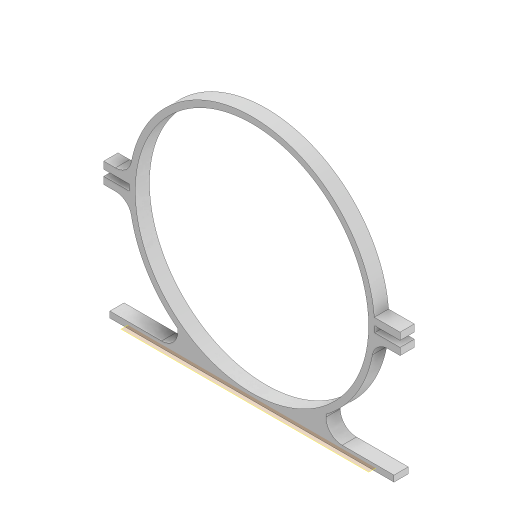
# Autodesk Inventor part: EXTRA_PARA CORTE DE TUBO
Saved by Autodesk Inventor 2024 (Build 280153000, 153)
## iProperties
Created: 2024-06-20
Part Number: EXTRA_PARA CORTE DE TUBO
Material: Generic
Document SubType Name: Modeling
Designer: Jhuliams
Density: 1 g/cm^3
Appearance: Default
Author: Jhuliams
Autodesk Inventor part; units mm, degrees
ref_plane "YZ Plane" through (0, 0, 0) normal (1, 0, 0) x (0, 1, 0)
ref_plane "XY Plane" through (0, 0, 0) normal (0, 0, 1) x (1, 0, 0)
sketch "Sketch1" plane through (0, 0, 0) normal (0, 0, 1) x (1, 0, 0)
  circle A0 centre (0, 0) radius 57.5
  circle A1 centre (0, 0) radius 60.5
  dimension "d0" = 115
  dimension "d1" = 121
  constraints: 2 centre point, 2 coincident
  measures "d0" diameter of A0
  measures "d1" diameter of A1
extrude "Extrusion1" add sketch "Sketch1" along normal blind 7
ref_plane "Work Plane1" through (0, -59, 0) normal (0, 1, 0) x (-1, 0, 0)
sketch "Sketch2" plane through (0, -59, 0) normal (0, 1, 0) x (-1, 0, 0)
  point P0 (0, 0)
sketch "Sketch3" plane through (0, -59, 0) normal (0, 1, 0) x (-1, 0, 0)
  line L0 (0, 0) -> (-70, 0)
  line L1 (-70, 0) -> (-70, 7)
  line L2 (-70, 7) -> (0, 7)
  line L3 (0, 7) -> (0, 0)
  line L4 (0, 0) -> (70, 0)
  line L5 (70, 0) -> (70, 7)
  line L6 (70, 7) -> (0, 7)
  dimension "d5" = 70
  dimension "d6" = 7
  constraints: 14 end point, 2 parallel, 2 symmetric about line, 1 horizontal, 1 perpendicular
  measures "d5" distance of L1.end L2.end
  measures "d6" distance of L0.end L1.end
extrude "Extrusion2" add sketch "Sketch3" along normal mid plane 3
sketch "Sketch4" plane through (0, 0, 7) normal (0, 0, 1) x (1, 0, 0)
  line L0 (48, 5) -> (73, 5)
  line L1 (73, 5) -> (73, -5)
  line L2 (73, -5) -> (48, -5)
  line L3 (48, -5) -> (48, 5)
  line L4 (48, 5) -> (73, -5) construction
  line L5 (73, 5) -> (48, -5) construction
  line L6 (48, 1.5) -> (73, 1.5)
  line L7 (73, 1.5) -> (73, -1.5)
  line L8 (73, -1.5) -> (48, -1.5)
  line L9 (48, -1.5) -> (48, 1.5)
  line L10 (48, 1.5) -> (73, -1.5) construction
  line L11 (73, 1.5) -> (48, -1.5) construction
  line L12 (0, 0) -> (0, -12.7)
  line L13 (-48, 5) -> (-73, 5)
  line L14 (-73, 5) -> (-73, -5)
  line L15 (-73, -5) -> (-48, -5)
  line L16 (-48, -5) -> (-48, 5)
  line L17 (-48, 5) -> (-73, -5) construction
  line L18 (-73, 5) -> (-48, -5) construction
  line L19 (-48, 1.5) -> (-73, 1.5)
  line L20 (-73, 1.5) -> (-73, -1.5)
  line L21 (-73, -1.5) -> (-48, -1.5)
  line L22 (-48, -1.5) -> (-48, 1.5)
  line L23 (-48, 1.5) -> (-73, -1.5) construction
  line L24 (-73, 1.5) -> (-48, -1.5) construction
  line L25 (-70, -60.5) -> (70, -60.5) projected
  line L26 (36.5, -75) -> (-36.5, -75)
  line L27 (-36.5, -75) -> (-36.5, -46)
  line L28 (-36.5, -46) -> (36.5, -46)
  line L29 (36.5, -46) -> (36.5, -75)
  line L30 (36.5, -75) -> (-36.5, -46) construction
  line L31 (-36.5, -75) -> (36.5, -46) construction
  line L32 (36.5, -60.5) -> (-36.5, -60.5)
  arc A0 (60.293, -5) -> (60.293, 5) centre (0, 0) ccw
  arc A1 (-60.293, 5) -> (-60.293, -5) centre (0, 0) ccw
  arc A2 (-36.5, -48.2494) -> (36.5, -48.2494) centre (0, 0) ccw
  point P0 (60.5, 0)
  point P1 (60.5, 0)
  point P2 (-60.5, 0)
  point P3 (-60.5, 0)
  point P4 (0, -60.5)
  point P5 (-60.4814, -1.5)
  point P6 (-60.4814, 1.5)
  point P7 (0, -60.5)
  point P8 (60.4814, -1.5)
  point P9 (60.4814, 1.5)
  dimension "d10" = 25
  dimension "d11" = 10
  dimension "d12" = 25
  dimension "d13" = 3
  dimension "d17" = 73
  dimension "d18" = 29
  constraints: 64 end point, 10 midpoint, 10 symmetric about line, 7 point on circle, 6 parallel, 6 point on line, 3 centre point, 3 horizontal, 3 perpendicular, 1 coincident, 1 vertical
  measures "d10" distance of L1.end L2.end
  measures "d11" distance of L0.end L1.end
  measures "d12" distance of L7.end L8.end
  measures "d13" distance of L6.end L7.end
  measures "d17" distance of L27.end L28.end
  measures "d18" distance of L26.end L27.end
extrude "Extrusion3" add sketch "Sketch4" against normal blind 7 contours L0 L1 L6 A0 | L8 L1 L2 A0 | A1 L19 L14 L13 | A1 L15 L14 L21 | L27 A2 L25 | A2 L29 L25
fillet "Fillet1" radius 8 5 edges at (-60.293, -5, 3.5) (-60.293, 5, 3.5) (60.293, -5, 3.5) (36.5, -57.5, 3.5) (-36.5, -57.5, 3.5)
body "Solid1"
